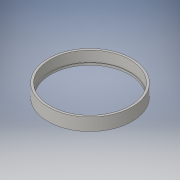
# Autodesk Inventor part: Adapter
Saved by Autodesk Inventor 2016 (Build 200138000, 138)
## iProperties
Created: 2015-08-14
Part Number: Adapter
Material: Generic
Document SubType Name: Modeling
Designer: Sudhar
Density: 1 g/cm^3
Appearance: Default
Author: Sudhar
Autodesk Inventor part; units mm, degrees
ref_plane "YZ Plane" through (0, 0, 0) normal (1, 0, 0) x (0, 1, 0)
ref_plane "XZ Plane" through (0, 0, 0) normal (0, 1, 0) x (-1, 0, 0)
ref_plane "XY Plane" through (0, 0, 0) normal (0, 0, 1) x (1, 0, 0)
sketch "Sketch1" plane through (0, 0, 0) normal (0, 1, 0) x (-1, 0, 0)
  circle A0 centre (0, 0) radius 25.4
  dimension "d0" = 50.8
  constraints: 1 centre point, 1 coincident
  measures "d0" diameter of A0
extrude "Extrusion1" add sketch "Sketch1" along normal blind 17.78
shell "Shell1" thickness 1.27 removed faces 1 at (7.2508, 17.78, -1.9085)
sketch "Sketch2" plane through (0, 0, 0) normal (0, -1, 0) x (1, 0, 0)
  circle A0 centre (0, 0) radius 22.86
  dimension "d4" = 45.72
  constraints: 1 centre point, 1 coincident
  measures "d4" diameter of A0
extrude "Extrusion2" cut sketch "Sketch2" against normal blind 7.62
sketch "Sketch4" plane through (0, 17.78, 0) normal (0, 1, 0) x (1, 0, 0)
  circle A0 centre (0, 0) radius 25.4
  circle A1 centre (0, 0) radius 24.13
  constraints: 2 centre point, 2 coincident
extrude "Extrusion4" cut sketch "Sketch4" against normal blind 10.16
sketch "Sketch5" plane through (0, 1.27, 0) normal (0, 1, 0) x (1, 0, 0)
  circle A0 centre (0, 0) radius 23.7732
  circle A1 centre (0, 0) radius 22.86
  constraints: 2 centre point, 2 coincident
extrude "Extrusion5" cut sketch "Sketch5" against normal blind 7.62
body "Solid1"
